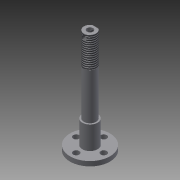
# Autodesk Inventor part: shaft
Saved by Autodesk Inventor 2015 SP1 (Build 190203100, 203)
## iProperties
Created: 2015-04-17
Part Number: shaft
Material: Ogólny
Document SubType Name: Modeling
Designer: Marcin
Density: 1 g/cm^3
Appearance: Domyślna
Author: Marcin
Autodesk Inventor part; units mm, degrees
ref_plane "YZ Plane" through (0, 0, 0) normal (1, 0, 0) x (0, 1, 0)
ref_plane "XZ Plane" through (0, 0, 0) normal (0, 1, 0) x (-1, 0, 0)
ref_plane "XY Plane" through (0, 0, 0) normal (0, 0, 1) x (1, 0, 0)
sketch "Szkic1" plane through (0, 0, 0) normal (0, 0, 1) x (1, 0, 0)
  circle A0 centre (0, 0) radius 13
  dimension "d0" = 26
  constraints: 1 centre point, 1 coincident
  measures "d0" diameter of A0
extrude "Wyciągnięcie proste1" add sketch "Szkic1" along normal blind 3
sketch "Szkic2" plane through (0, 0, 3) normal (0, 0, 1) x (1, 0, 0)
  circle A0 centre (0, 0) radius 5
  dimension "d3" = 10
  constraints: 1 centre point, 1 coincident
  measures "d3" diameter of A0
extrude "Wyciągnięcie proste2" add sketch "Szkic2" along normal blind 15
sketch "Szkic3" plane through (0, 0, 18) normal (0, 0, 1) x (1, 0, 0)
  circle A0 centre (0, 0) radius 4
  dimension "d6" = 8
  constraints: 1 centre point, 1 coincident
  measures "d6" diameter of A0
extrude "Wyciągnięcie proste3" add sketch "Szkic3" along normal blind 50
thread "Gwint1" size "M8x1.25" class "6g" standard "ANSI Metric M Profile" length 20
sketch "Szkic4" plane through (0, 0, 68) normal (0, 0, 1) x (1, 0, 0)
  circle A0 centre (0, 0) radius 2
  dimension "d11" = 4
  constraints: 2 coincident, 1 centre point
  measures "d11" diameter of A0
sketch "Szkic9" plane through (0, 0, 68) normal (0, 0, 1) x (1, 0, 0)
  circle A0 centre (0, 0) radius 4 projected
  line L0 (-1.9365, 3.5) -> (1.9365, 3.5)
  dimension "d34" = 3.5
  constraints: 2 end point, 2 point on circle, 1 horizontal
  measures "d34" distance from line of L0 point (0, 0)
extrude "Wyciągnięcie proste7" cut sketch "Szkic9" against normal blind 5 contours L0 A0 picked at (-0.3981, 3.6058)
sketch "Szkic10" plane through (-1.9365, 3.5, 68) normal (0, 1, 0) x (1, 0, 0)
  line L0 (3.873, 0) -> (0, 0) projected
  line L1 (3.873, 5) -> (3.873, 0) projected
  line L2 (3.873, 5) -> (0, 5) projected
  line L3 (0, 0) -> (0, 5) projected
  line L4 (3.873, 5) -> (3.873, 0) construction
  line L5 (3.873, 2.5) -> (0, 2.5) construction
  line L6 (0, 0) -> (0, 5) construction
  point P0 (1.9365, 68)
  point P1 (1.9365, 2.5)
  constraints: 3 midpoint, 2 end point
hole "Otwór2" at (0, 3.5, 65.5) direction (0, -1, 0) diameter 3 depth 20 tip angle 118
hole "Otwór3" at (0, 0, 68) direction (0, 0, -1) diameter 4 depth 11 tip angle 118
sketch "Szkic11" plane through (0, 0, 0) normal (0, 0, -1) x (-1, 0, 0)
  circle A0 centre (0, 0) radius 9 construction
  line L0 (9, 0) -> (-9, 0) construction
  line L1 (0, -9) -> (0, 9) construction
  dimension "d55" = 18
  constraints: 4 end point, 4 point on circle, 3 midpoint, 1 centre point, 1 coincident, 1 horizontal, 1 vertical
  measures "d55" diameter of A0
hole "Otwór4" at (9, 0, 0) at (-9, 0, 0) at (0, -9, 0) at (0, 9, 0) direction (0, 0, 1) diameter 4 depth 8 tip angle 118
thread "Gwint3" size "M3x0.5" class "6H" standard "ANSI Metric M Profile" full length
thread "Gwint4" size "M3x0.5" class "6H" standard "ANSI Metric M Profile" full length
